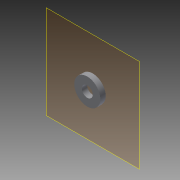
# Autodesk Inventor part: gearSpacerSmallOutputStage
Saved by Autodesk Inventor 2013 (Build 170138000, 138)
## iProperties
Created: 2014-07-01
Part Number: gearSpacerSmallOutputStage
Material: Generic
Document SubType Name: Modeling
Designer: Nano
Density: 1 g/cm^3
Author: Nano
Autodesk Inventor part; units mm, degrees
ref_plane "YZ Plane" through (0, 0, 0) normal (1, 0, 0) x (0, 1, 0)
ref_plane "XZ Plane" through (0, 0, 0) normal (0, 1, 0) x (-1, 0, 0)
ref_plane "XY Plane" through (0, 0, 0) normal (0, 0, 1) x (1, 0, 0)
ref_plane "Work Plane1" through (-85.4591, -7.5098, 0) normal (0, 0, 1) x (0.9989, 0.0477, 0)
sketch "Sketch1" plane through (-85.4591, -7.5098, 0) normal (0, 0, 1) x (0.9989, 0.0477, 0)
  circle A0 centre (85.7201, 3.4229) radius 3.175 projected
  circle A1 centre (85.7201, 3.4229) radius 7.62
  point P0 (85.7201, 3.4229)
  dimension "d0" = 15.24
  constraints: 1 centre point
  measures "d0" diameter of A1
extrude "Extrusion1" add sketch "Sketch1" along normal blind 3.175
body "Solid1"
